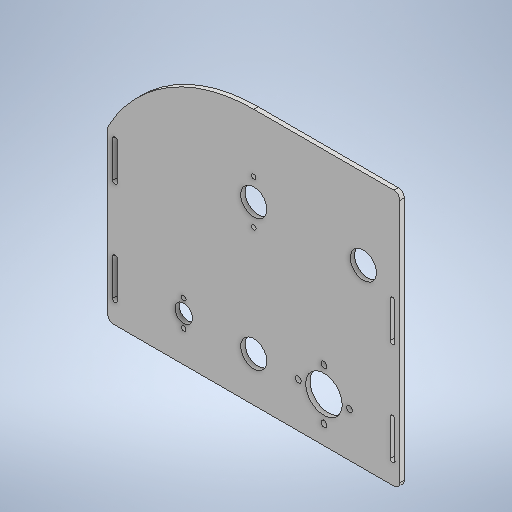
# Autodesk Inventor part: aaa_small_plate_motor
Saved by Autodesk Inventor 2025.1 (Build 291241000, 241)
## iProperties
Created: 2024-12-20
Part Number: aaa_small_plate_motor
Material: 一般
Document SubType Name: Modeling
Designer: yuki0520
Density: 1 g/cm^3
Appearance: 既定
Author: yuki0520
Autodesk Inventor part; units mm, degrees
ref_plane "YZ Plane" through (0, 0, 0) normal (1, 0, 0) x (0, 1, 0)
ref_plane "XZ Plane" through (0, 0, 0) normal (0, 1, 0) x (-1, 0, 0)
ref_plane "XY Plane" through (0, 0, 0) normal (0, 0, 1) x (1, 0, 0)
sketch "スケッチ1" plane through (0, 0, 0) normal (0, 0, 1) x (1, 0, 0)
  point P0 (0, 0)
sketch "スケッチ2" plane through (0, 0, 0) normal (0, 0, 1) x (1, 0, 0)
  line L0 (100, -52.5) -> (-100, -52.5)
  line L1 (-100, -52.5) -> (-100, 52.5)
  line L2 (-100, 52.5) -> (100, 52.5)
  line L3 (100, 52.5) -> (100, -52.5)
  line L4 (100, -52.5) -> (-100, 52.5) construction
  line L5 (-100, -52.5) -> (100, 52.5) construction
  circle A0 centre (-48, -32) radius 6.05
  circle A1 centre (48, -32) radius 12.55
  circle A2 centre (48, -32) radius 17.5
  circle A3 centre (65.5, -32) radius 2.05
  circle A4 centre (48, -14.5) radius 2.05
  circle A5 centre (30.5, -32) radius 2.05
  circle A6 centre (48, -49.5) radius 2.05
  circle A7 centre (-48, -32) radius 9
  circle A8 centre (-57, -32) radius 1.6
  circle A9 centre (-48, -41) radius 1.6
  circle A10 centre (-39, -32) radius 1.6
  circle A11 centre (-48, -23) radius 1.6
  line L6 (95, 47.5) -> (-95, 47.5)
  line L7 (-95, 47.5) -> (-95, -47.5)
  line L8 (-95, -47.5) -> (95, -47.5)
  line L9 (95, -47.5) -> (95, 47.5)
  line L10 (-95, 47.5) -> (-95, 22.5) construction
  line L11 (-96.6, 47.5) -> (-96.6, 22.5)
  line L12 (-93.4, 22.5) -> (-93.4, 47.5)
  arc A12 (-93.4, 47.5) -> (-96.6, 47.5) centre (-95, 47.5) ccw
  arc A13 (-96.6, 22.5) -> (-93.4, 22.5) centre (-95, 22.5) ccw
  line L13 (-95, 47.5) -> (-70, 47.5) construction
  line L14 (-95, -47.5) -> (-95, -22.5) construction
  line L15 (-93.4, -47.5) -> (-93.4, -22.5)
  line L16 (-96.6, -22.5) -> (-96.6, -47.5)
  arc A14 (-96.6, -47.5) -> (-93.4, -47.5) centre (-95, -47.5) ccw
  arc A15 (-93.4, -22.5) -> (-96.6, -22.5) centre (-95, -22.5) ccw
  line L17 (-95, -47.5) -> (-70, -47.5) construction
  line L18 (95, 47.5) -> (95, 22.5) construction
  line L19 (93.4, 47.5) -> (93.4, 22.5)
  line L20 (96.6, 22.5) -> (96.6, 47.5)
  arc A16 (96.6, 47.5) -> (93.4, 47.5) centre (95, 47.5) ccw
  arc A17 (93.4, 22.5) -> (96.6, 22.5) centre (95, 22.5) ccw
  line L21 (95, 47.5) -> (120, 47.5) construction
  line L22 (95, -47.5) -> (95, -22.5) construction
  line L23 (96.6, -47.5) -> (96.6, -22.5)
  line L24 (93.4, -22.5) -> (93.4, -47.5)
  arc A18 (93.4, -47.5) -> (96.6, -47.5) centre (95, -47.5) ccw
  arc A19 (96.6, -22.5) -> (93.4, -22.5) centre (95, -22.5) ccw
  line L25 (95, -47.5) -> (120, -47.5) construction
  line L26 (-100, -32) -> (100, -32)
  circle A20 centre (0, -32) radius 9
  circle A21 centre (0, -32) radius 39
  line L27 (-85, 52.5) -> (85, 52.5)
  line L28 (85, 52.5) -> (85, 47.5)
  line L29 (85, 47.5) -> (-85, 47.5)
  line L30 (-85, 47.5) -> (-85, 52.5)
  line L31 (-85, 47.5) -> (0, 0)
  line L32 (0, 0) -> (85, 47.5)
  line L33 (-100, 0) -> (100, 0)
  line L34 (100, 0) -> (100, -62.5)
  line L35 (100, -62.5) -> (-100, -62.5)
  line L36 (-100, -62.5) -> (-100, 0)
  arc A22 (100, 52.5) -> (-100, 52.5) centre (0, 0) ccw
  circle A23 centre (0, 58) radius 15
  line L37 (0, 112.9436) -> (0, -32)
  circle A24 centre (0, 58) radius 9
  circle A25 centre (0, 73) radius 1.55
  circle A26 centre (0, 43) radius 1.55
  circle A27 centre (75, 58) radius 9
  circle A28 centre (75, 58) radius 24
  circle A29 centre (0, -32) radius 24
  line L38 (-15, 58) -> (15, 58)
  line L39 (-100, 52.5) -> (100, 52.5)
  line L40 (100, 52.5) -> (100, 112.9436)
  line L41 (100, 112.9436) -> (-100, 112.9436)
  line L42 (-100, 112.9436) -> (-100, 52.5)
  point P0 (-95, 35)
  point P1 (-95, -35)
  point P2 (95, 35)
  point P3 (95, -35)
  point P4 (-39.1422, -33.5937)
  point P5 (-39.1422, -30.4063)
  point P6 (0, 52.5)
  point P7 (85, 52.5)
  point P8 (48.45, -47.5)
  point P9 (47.55, -47.5)
  dimension "d9" = 35
  dimension "d15" = 18
  dimension "d0" = 200
  dimension "d1" = 105
  dimension "d5" = 12.1
  dimension "d6" = 25.1
  dimension "d10" = 4.1
  dimension "d13" = 360
  dimension "d16" = 3.2
  dimension "d19" = 360
  dimension "d21" = 5
  dimension "d22" = 25
  dimension "d23" = 90
  dimension "d24" = 3.2
  dimension "d25" = 25
  dimension "d26" = 90
  dimension "d27" = 3.2
  dimension "d28" = 25
  dimension "d29" = 90
  dimension "d30" = 3.2
  dimension "d31" = 25
  dimension "d32" = 90
  dimension "d33" = 3.2
  dimension "d36" = 20.5
  dimension "d37" = 18
  dimension "d38" = 78
  dimension "d39" = 48
  dimension "d40" = 48
  dimension "d43" = 170
  dimension "d44" = 85
  dimension "d46" = 62.5
  dimension "d47" = 30
  dimension "d49" = 18
  dimension "d50" = 3.1
  dimension "d51" = 3.1
  dimension "d52" = 18
  dimension "d53" = 48
  dimension "d54" = 48
  dimension "d56" = 90
  dimension "d57" = 75
  constraints: 94 end point, 28 centre point, 23 point on circle, 17 tangent, 14 parallel, 12 point on line, 11 perpendicular, 10 midpoint, 8 horizontal, 6 coincident, 6 collinear, 1 concentric, 1 horizontal alignment, 1 vertical, 26 other
  measures "d0" distance of L1.end L2.end
  measures "d1" distance of L0.end L1.end
  measures "d5" diameter of A0
  measures "d6" diameter of A1
  measures "d10" diameter of A3
  measures "d16" diameter of A8
  measures "d21" distance between parallel lines of L2 L6
  measures "d22" distance of L6.end L10.end
  measures "d23" angle of L10 L13
  measures "d24" diameter of A13
  measures "d25" distance of L7.end L14.end
  measures "d26" angle of L17 L14
  measures "d27" diameter of A15
  measures "d28" distance of L6.start L18.end
  measures "d29" angle of L18 L21
  measures "d30" diameter of A17
  measures "d31" distance of L8.end L22.end
  measures "d32" angle of L25 L22
  measures "d33" diameter of A19
  measures "d36" distance between parallel lines of L0 L26
  measures "d37" diameter of A20
  measures "d38" diameter of A21
  measures "d39" distance of A1.centre A20.centre
  measures "d40" distance of A0.centre A20.centre
  measures "d43" distance of L28.end L29.end
  measures "d44" distance from line of point (0, 52.5) L30
  measures "d46" distance of L33.end L34.end
  measures "d47" diameter of A23
  measures "d49" diameter of A24
  measures "d50" diameter of A25
  measures "d51" diameter of A26
  measures "d52" diameter of A27
  measures "d53" diameter of A28
  measures "d54" diameter of A29
  measures "d56" distance of L37.end A23.centre
  measures "d57" distance of A23.centre A28.centre
extrude "押し出し1" add sketch "スケッチ2" along normal blind 3 contours L34 L35 A21 L0 | L0 A21 L8 A2 A6 A18 L23 L26 L3 | A21 L35 L0 A29 | L0 A29 L8 A21 | L26 L23 A19 L9 L33 L3 | A29 L0 | L0 A29 L8 | A21 A2 L8 | L8 A29 L26 A5 A2 A21 | L33 L9 A17 L20 A16 A28 L2 L3 | L0 A21 L8 A29 | L8 A29 L26 A20 | L35 L36 L0 A21 | L8 A6 A2 | A2 A21 A1 L26 A3 L8 A6 | A2 A5 L26 A1 A21 | L2 A28 A22 | A22 A28 L41 L40 | L33 A21 L32 A28 L19 A17 L9 | L9 A19 L24 L26 A3 A2 A4 A21 L33 | L0 L1 L26 L16 A14 L8 A21 | L8 A21 A10 L26 A29 | A29 L37 L33 A21 A2 A5 L26 | L26 A20 L37 A29 | A6 L8 | A28 A16 L6 L28 L2 | L2 A27 A28 A22 | A22 A28 | L33 L32 A21 | L8 A2 A3 L26 L24 | L8 L15 L26 A8 A7 A9 A10 A21 | A29 L37 A20 L26 | L26 A10 A21 L33 L37 A29 | A6 L8 A2 | A5 A2 A21 A1 L26 | A1 A21 A2 A4 A3 L26 | L28 L6 A28 L2 A27 | A28 L2 A23 A25 L37 A22 | L37 A25 A23 L2 A22 | L32 L37 A21 | A21 L37 A26 A23 L6 A28 L32 | L33 A21 L31 | L31 A21 L37 | L1 L33 L7 A15 L16 L26 | A21 L26 A10 | A10 A7 A21 | L26 A21 A10 | L32 A28 L6 | L6 L19 A28 L32 | A28 L6 A23 L2 | L2 L30 L6 A12 L11 A13 L7 L33 L1 | A21 L31 L6 A23 A26 L37 | A21 L33 L7 A13 L12 L6 L31 | A21 A10 A7 A11 A8 L26 L15 A15 L7 L33 | A10 L26 A7 | A7 A9 A8 L26 A0 A10 | L26 A10 A7 | A7 A10 A21 | A23 L6 L37 A24 L2 | L2 A24 L38 A23 | L2 A23 L6 L30 | A25 L37 A24 L38 A23 | L26 A7 A8 | A8 A7 L26 | L26 A0 A8 A7 A11 A10 | A23 A26 L37 L6 | L38 A24 L37 A25 A23 | A23 L38 A24 L2 | L2 A24 L37 L6 A23 | A23 L6 L37 A26 | A8 L26 A7 | A7 L26 A8 picked at (42.8176, -47.9142) picked at (53.1824, -47.9142)
fillet "フィレット1" radius 4 4 edges at (-100, 52.5, 1.5) (100, -62.5, 1.5) (-100, -62.5, 1.5) (100, 112.9436, 1.5)
equation "\"d25\" = d22"
equation "\"d27\" = d24"
equation "\"d28\" = d22"
equation "\"d30\" = d24"
equation "\"d31\" = d22"
equation "\"d33\" = d24"
equation "\"d40\" = d39"
equation "\"d44\" = 0.5 * d43"
